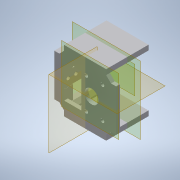
# Autodesk Inventor part: 30_Cube_Z_Focus_NEMA8_captive_base_v0
Saved by Autodesk Inventor 2022 (Build 260153000, 153)
## iProperties
Created: 2021-04-25
Part Number: 30_Cube_Z_Focus_NEMA8_captive_base_v0
Material: Generic
Document SubType Name: Modeling
Designer: diederichbenedict
Density: 1 g/cm^3
Appearance: Smooth - White
Author: diederichbenedict
Autodesk Inventor part; units mm, degrees
ref_plane "Work Plane1" through (0, 0, 13.5808) normal (0, 0, -1) x (-1, 0, 0)
sketch "Sketch1" plane through (0, 0, 13.5808) normal (0, 0, -1) x (-1, 0, 0)
  line L0 (24.85, 16.87) -> (16.87, 16.87)
  line L1 (16.87, -16.87) -> (24.85, -16.87)
  line L2 (24.85, -16.87) -> (24.85, 16.87)
  line L3 (-16.87, 24.85) -> (16.87, 24.85)
  line L4 (16.87, 24.85) -> (16.87, 13.87)
  line L5 (16.87, 13.87) -> (-16.87, 13.87)
  line L6 (-16.87, 13.87) -> (-16.87, 24.85)
  line L7 (-16.87, 16.87) -> (-24.85, 16.87)
  line L8 (-24.85, 16.87) -> (-24.85, -16.87)
  line L9 (-24.85, -16.87) -> (-16.87, -16.87)
  line L10 (-16.87, -24.85) -> (16.87, -24.85)
  line L11 (16.87, -24.85) -> (16.87, -13.87)
  line L12 (16.87, -13.87) -> (-16.87, -13.87)
  line L13 (-16.87, -13.87) -> (-16.87, -24.85)
  circle A0 centre (-22.53, 11.5) radius 1.025 construction
  circle A1 centre (-22.53, -11.5) radius 1.025 construction
  line L14 (-11.03, -14.1) -> (-11.03, -12.75) construction
  arc A2 (-11.03, 12.75) -> (-11.03, -12.75) centre (-11.03, 0) ccw construction
  line L15 (-11.03, 12.75) -> (-11.03, 14.1) construction
  line L16 (-11.03, 14.1) -> (-22.53, 14.1) construction
  arc A3 (-22.53, 14.1) -> (-25.13, 11.5) centre (-22.53, 11.5) ccw construction
  line L17 (-25.13, 11.5) -> (-25.13, -11.5) construction
  arc A4 (-25.13, -11.5) -> (-22.53, -14.1) centre (-22.53, -11.5) ccw construction
  line L18 (-22.53, -14.1) -> (-11.03, -14.1) construction
  circle A5 centre (-11.03, 0) radius 12.75 construction
  circle A6 centre (0.47, 11.5) radius 1.025 construction
  circle A7 centre (0.47, -11.5) radius 1.025 construction
  circle A8 centre (-22.53, -11.5) radius 1.025 construction
  circle A9 centre (-22.53, 11.5) radius 1.025 construction
  line L19 (-22.53, -14.1) -> (0.47, -14.1) construction
  arc A10 (-25.13, -11.5) -> (-22.53, -14.1) centre (-22.53, -11.5) ccw construction
  line L20 (-25.13, 11.5) -> (-25.13, -11.5) construction
  arc A11 (-22.53, 14.1) -> (-25.13, 11.5) centre (-22.53, 11.5) ccw construction
  line L21 (0.47, 14.1) -> (-22.53, 14.1) construction
  arc A12 (3.07, 11.5) -> (0.47, 14.1) centre (0.47, 11.5) ccw construction
  line L22 (3.07, -11.5) -> (3.07, 11.5) construction
  arc A13 (0.47, -14.1) -> (3.07, -11.5) centre (0.47, -11.5) ccw construction
  line L23 (-16.87, 13.87) -> (3.07, 13.87)
  line L24 (3.07, 13.87) -> (3.07, -13.87)
  line L25 (3.07, -13.87) -> (-16.87, -13.87)
  line L26 (16.87, 6.05) -> (16.8476, 6.05)
  line L27 (16.8476, 6.05) -> (16.8476, -6.05)
  line L28 (16.8476, -6.05) -> (16.87, -6.05)
  line L29 (16.87, -6.05) -> (16.87, -4.7)
  line L30 (16.87, 4.7) -> (16.87, 6.05)
  line L31 (16.87, 16.87) -> (16.87, 6.05)
  line L32 (16.87, -6.05) -> (16.87, -16.87)
  line L33 (5.6476, 13.2) -> (13.4476, 13.2) projected
  line L34 (13.4476, -13.2) -> (5.6476, -13.2) projected
  circle A14 centre (-4.7031, 0) radius 7 construction
  circle A15 centre (-4.7031, 0) radius 4 construction
  point P0 (0, 0)
  point P1 (16.87, 16.87)
  point P2 (3.07, 13.87)
  point P3 (3.07, 13.87)
  point P4 (-16.87, -16.87)
  dimension "d6" = 3
  dimension "d7" = 3
  dimension "d140" = 8
  constraints: 48 end point, 12 parallel, 7 perpendicular, 6 horizontal, 6 point on line, 2 centre point, 1 coincident, 2 other
  measures "d6" distance between parallel lines of L7 L5
  measures "d7" distance between parallel lines of L9 L12
  measures "d140" diameter of A15
extrude "Extrusion1" add sketch "Sketch1" along normal blind 3 contours L2 L1 L11 L32 L28 L27 L26 L31 L4 L0 | L4 L5 L6 L3 | L11 L10 L13 L12 | L24 L12 L13 L9 L8 L7 L6 L5
chamfer "Chamfer1" distance 3.9 angle 45 4 edges at (-16.87, -16.87, 12.0808) (16.87, -16.87, 12.0808) (16.87, 16.87, 12.0808) (-16.87, 16.87, 12.0808)
sketch "Sketch2" plane through (0, 0, 10.5808) normal (0, 0, -1) x (-1, 0, 0)
  line L0 (3.07, 13.87) -> (16.87, 13.87) projected
  line L1 (16.87, -13.87) -> (3.07, -13.87) projected
  line L2 (-16.87, -20.77) -> (-16.87, -24.85) construction
  line L3 (-16.87, -24.85) -> (16.87, -24.85) construction
  line L4 (16.87, -6.05) -> (16.87, -13.87) projected
  line L5 (16.87, 20.77) -> (16.87, 24.85) construction
  line L6 (16.87, 24.85) -> (-16.87, 24.85) construction
  line L7 (-16.87, 24.85) -> (-16.87, 20.77) construction
  line L8 (-13.8689, -21.8489) -> (-13.8689, -19.5269)
  line L9 (-13.8689, -19.5269) -> (-19.5269, -13.8689)
  line L10 (-19.5269, -13.8689) -> (-21.8489, -13.8689)
  line L11 (-21.8489, 13.8689) -> (-19.5269, 13.8689)
  line L12 (-19.5269, 13.8689) -> (-13.8689, 19.5269)
  line L13 (-13.8689, 19.5269) -> (-13.8689, 21.8489)
  line L14 (-13.8689, 21.8489) -> (-13.8689, 24.85)
  line L15 (-21.8489, 13.8689) -> (-24.85, 13.8689)
  line L16 (-21.8489, -13.8689) -> (-24.85, -13.8689)
  line L17 (-13.8689, -21.8489) -> (-13.8689, -24.85)
  line L18 (-11.5469, -21.8489) -> (-13.8689, -21.8489)
  line L19 (-21.8489, -13.8689) -> (-21.8489, -11.5469)
  line L20 (-21.8489, 11.5469) -> (-21.8489, 13.8689)
  line L21 (-13.8689, 21.8489) -> (-11.5469, 21.8489)
  line L22 (16.87, 13.87) -> (16.87, 6.05) projected
  line L23 (16.87, 6.05) -> (16.8476, 6.05) projected
  line L24 (16.8476, 6.05) -> (16.8476, -6.05) projected
  line L25 (16.8476, -6.05) -> (16.87, -6.05) projected
  line L26 (20.77, -16.87) -> (24.85, -16.87) construction
  line L27 (24.85, -16.87) -> (24.85, 16.87) construction
  line L28 (24.85, 16.87) -> (20.77, 16.87) construction
  line L29 (16.87, 20.77) -> (20.77, 16.87) construction
  line L30 (16.87, -24.85) -> (16.87, -20.77) construction
  line L31 (20.77, -16.87) -> (16.87, -20.77) construction
  line L32 (-13.87, 21.85) -> (13.87, 21.85) construction
  line L33 (13.87, 21.85) -> (13.87, 19.5274) construction
  line L34 (13.87, 19.5274) -> (19.5274, 13.87) construction
  line L35 (19.5274, 13.87) -> (21.85, 13.87) construction
  line L36 (21.85, 13.87) -> (21.85, -13.87) construction
  line L37 (21.85, -13.87) -> (19.5274, -13.87) construction
  line L38 (19.5274, -13.87) -> (13.87, -19.5274) construction
  line L39 (13.87, -19.5274) -> (13.87, -21.85) construction
  line L40 (13.87, -21.85) -> (-13.87, -21.85) construction
  line L41 (-13.87, -21.85) -> (-13.87, -19.5274) construction
  line L42 (-13.87, -19.5274) -> (-19.5274, -13.87) construction
  line L43 (-19.5274, -13.87) -> (-21.85, -13.87) construction
  line L44 (-21.85, -13.87) -> (-21.85, 13.87) construction
  line L45 (-21.85, 13.87) -> (-19.5274, 13.87) construction
  line L46 (-19.5274, 13.87) -> (-13.87, 19.5274) construction
  line L47 (-13.87, 19.5274) -> (-13.87, 21.85) construction
  line L48 (16.87, 24.85) -> (-16.87, 24.85) projected
  line L49 (13.87, 24.85) -> (13.87, 19.5274)
  line L50 (13.87, 19.5274) -> (19.5274, 13.87)
  line L51 (19.5274, 13.87) -> (24.85, 13.87)
  line L52 (24.85, -16.87) -> (24.85, 16.87) projected
  line L53 (24.85, -13.87) -> (19.5274, -13.87)
  line L54 (19.5274, -13.87) -> (13.87, -19.5274)
  line L55 (-16.87, -24.85) -> (16.87, -24.85) projected
  line L56 (13.87, -24.85) -> (13.87, -19.5274)
  line L57 (16.87, 24.85) -> (-16.87, 24.85) projected
  line L58 (13.87, 24.85) -> (16.87, 24.85)
  line L59 (16.87, 24.85) -> (16.87, 20.77)
  line L60 (16.87, 20.77) -> (20.77, 16.87)
  line L61 (24.85, 16.87) -> (20.77, 16.87) projected
  line L62 (24.85, 16.87) -> (20.77, 16.87)
  line L63 (24.85, -16.87) -> (24.85, 16.87) projected
  line L64 (24.85, 16.87) -> (24.85, 13.87)
  line L65 (24.85, -13.87) -> (24.85, -16.87)
  line L66 (24.85, -16.87) -> (20.77, -16.87)
  line L67 (20.77, -16.87) -> (16.87, -20.77)
  line L68 (16.87, -24.85) -> (16.87, -20.77) projected
  line L69 (16.87, -24.85) -> (16.87, -20.77)
  line L70 (16.87, -20.77) -> (16.87, -24.85)
  line L71 (16.87, -24.85) -> (-16.87, -24.85) projected
  line L72 (13.87, -24.85) -> (16.87, -24.85)
  line L73 (3.07, -13.87) -> (3.07, 13.87) projected
  line L74 (-20.77, 16.87) -> (-24.85, 16.87) projected
  line L75 (-24.85, 16.87) -> (-24.85, -16.87) projected
  line L76 (-24.85, -16.87) -> (-20.77, -16.87) projected
  line L77 (-16.87, -20.77) -> (-20.77, -16.87) projected
  line L78 (-20.77, 16.87) -> (-16.87, 20.77) projected
  point P0 (0, 0)
  dimension "d115" = 3
  constraints: 94 end point, 14 point on line, 6 collinear, 5 perpendicular, 1 horizontal, 1 vertical, 9 other
  measures "d115" distance between parallel lines of L6 L32
ref_plane "Work Plane2" through (-16.97, -24.85, 34.1) normal (0, 0, -1) x (0, 1, 0)
extrude "Extrusion2" add sketch "Sketch2" along normal blind 31.5 contours L56 L54 L53 L52 L66 L67 L68 L55 | L51 L50 L49 L48 L59 L60 L61 L52
sketch "Sketch4" plane through (-24.85, -16.87, 13.5808) normal (-1, 0, 0) x (0, 0, 1)
  line L0 (37.9, 11.3739) -> (37.9, 18.453) construction
  line L1 (23.6194, 18.453) -> (37.9, 18.453) construction
  arc A0 (22.1806, 18.453) -> (23.6194, 18.453) centre (22.9, 16.8577) ccw construction
  line L2 (-1.3806, 18.453) -> (22.1806, 18.453) construction
  arc A1 (-2.8194, 18.453) -> (-1.3806, 18.453) centre (-2.1, 16.8577) ccw construction
  line L3 (-31.3806, 18.453) -> (-2.8194, 18.453) construction
  arc A2 (-32.8194, 18.453) -> (-31.3806, 18.453) centre (-32.1, 16.8577) ccw construction
  line L4 (-42.1, 18.453) -> (-32.8194, 18.453) construction
  line L5 (-42.1, 11.3739) -> (-42.1, 18.453) construction
  line L6 (-42.1, 11.3739) -> (37.9, 11.3739) construction
  line L7 (37.9, 19.2506) -> (37.9, 22.3415) construction
  line L8 (-42.1, 22.3415) -> (37.9, 22.3415) construction
  line L9 (-42.1, 19.2506) -> (-42.1, 22.3415) construction
  line L10 (-42.1, 19.2506) -> (37.9, 19.2506) construction
  line L11 (-3, 3) -> (-3, 30.74) construction
  line L12 (-34.1, 33.84) -> (-34.1, -5.98) construction
  line L13 (-3, 11.3739) -> (-34.1, 11.3739)
  line L14 (-34.1, 11.3739) -> (-34.1, 22.3415)
  line L15 (-34.1, 22.3415) -> (-3, 22.3415)
  line L16 (-3, 22.3415) -> (-3, 11.3739)
  line L17 (-34.1, 11.3739) -> (-32.1, 11.3739)
  line L18 (-32.1, 11.3739) -> (-32.1, 3.0011)
  line L19 (-32.1, 3.0011) -> (-34.1, 3.0011)
  line L20 (-34.1, 3.0011) -> (-34.1, 11.3739)
  line L21 (-34.1, 22.3415) -> (-32.1, 22.3415)
  line L22 (-32.1, 22.3415) -> (-32.1, 30.7389)
  line L23 (-32.1, 30.7389) -> (-34.1, 30.7389)
  line L24 (-34.1, 30.7389) -> (-34.1, 22.3415)
  point P0 (-13.5808, 16.87)
  point P1 (-3, 3.0011)
  point P2 (-3, 30.7389)
  point P3 (-3, 33.74)
  point P4 (-3, 31.418)
  point P5 (-3, 0)
  dimension "d24" = 2
  constraints: 24 end point, 6 parallel, 5 point on line, 3 horizontal, 3 perpendicular
  measures "d24" distance of L18.end L19.end
ref_plane "Work Plane3" through (16.97, -5.4961, -37.9) normal (1, 0, 0) x (0, 1, 0)
extrude "Extrusion4" add sketch "Sketch4" against normal blind 7.88 contours L13 L14 L15 L16
sketch "Sketch5" plane through (-24.85, -16.87, 13.5808) normal (-1, 0, 0) x (0, 0, 1)
  circle A0 centre (-32.1, 16.87) radius 1.4
  circle A1 centre (-3.4423, 16.87) radius 1.4
  line L0 (0, -7.98) -> (-34.5, -7.98) projected
  line L1 (0, 41.72) -> (-34.5, 41.72) projected
  line L2 (0, -7.98) -> (-34.5, -7.98) projected
  point P0 (-13.5808, 16.87)
  dimension "d25" = 2.8
  dimension "d26" = 2.8
  dimension "d86" = 49.7
  dimension "d87" = 24.85
  dimension "d88" = 0
  constraints: 2 centre point
  measures "d25" diameter of A0
  measures "d26" diameter of A1
  measures "d86" distance between parallel lines of L1 L2
  measures "d87" distance from line of A0.centre L1
  measures "d88" vertical distance of A1.centre A0.centre
extrude "Extrusion5" cut sketch "Sketch5" against normal blind 10
pattern_linear "Rectangular Pattern1" count 5 spacing 6.25 along (0, 0, -1) of "Extrusion5"
ref_plane "Work Plane4" through (-25.03, -12.97, -12) normal (0, 0, 1) x (1, 0, 0)
sketch "Sketch12" plane through (-24.85, -16.87, 13.5808) normal (-1, 0, 0) x (0, 0, 1)
  ellipse E0 centre (-17.053, 16.87) end of major axis (-32.053, 16.87) minor radius 10.6066 projected
  circle A0 centre (-32.1, 16.87) radius 1.4 projected
  circle A1 centre (-22.1923, 16.87) radius 1.4 projected
  circle A2 centre (-15.9423, 16.87) radius 1.4 projected
  circle A3 centre (-9.6923, 16.87) radius 1.4 projected
  circle A4 centre (-3.4423, 16.87) radius 1.4 projected
  circle A5 centre (-28.4423, 16.87) radius 1.4 projected
  point P0 (-13.5808, 16.87)
  constraints: 1 other
hole "Hole2" at (-24.85, 0, -8.6115) at (-24.85, 0, 3.8885) at (-24.85, 0, 10.1385) at (-24.85, 0, -2.3615) at (-24.85, 0, -14.8615) direction (1, 0, 0) diameter 2.8 depth 8 tip angle 118 counterbore diameter 6 counterbore depth 3
ref_plane "Work Plane6" through (0, 0, -22) normal (0, 0, -1) x (-1, 0, 0)
ref_plane "Work Plane5" through (-16.97, -16.97, 0) normal (0, 0, 1) x (1, 0, 0)
ref_plane "Work Plane7" through (0, -16.87, 13.5808) normal (1, 0, 0) x (0, 0, -1)
ref_plane "Work Plane8" through (16.87, 0, 13.5808) normal (0, 1, 0) x (-1, 0, 0)
sketch "Skizze18" plane through (-24.85, -16.87, 13.5808) normal (-1, 0, 0) x (0, 0, 1)
  line L0 (0, 0) -> (-34.5, 0) projected
  line L1 (0, 0) -> (0, 33.74) projected
  line L2 (0, 33.74) -> (-34.5, 33.74) projected
  arc A0 (-31.2335, 15.7704) -> (-31.2335, 17.9696) centre (-28.4423, 16.87) ccw projected
  arc A1 (-31.2335, 17.9696) -> (-31.2335, 15.7704) centre (-32.1, 16.87) ccw projected
  circle A2 centre (-3.4423, 16.87) radius 3 projected
  circle A3 centre (-22.1923, 16.87) radius 3 projected
  circle A4 centre (-9.6923, 16.87) radius 3 projected
  circle A5 centre (-15.9423, 16.87) radius 3 projected
  line L3 (-3, 30.7389) -> (-34.5, 30.7389) projected
  line L4 (-34.1, 30.7389) -> (-3, 30.7389)
  line L5 (-3, 30.7389) -> (-3, 33.74)
  line L6 (-3, 33.74) -> (-34.1, 33.74)
  line L7 (-34.1, 33.74) -> (-34.1, 30.7389)
  line L8 (-3, 3.0011) -> (-34.5, 3.0011) projected
  line L9 (0, 0) -> (-34.5, 0) projected
  line L10 (-3, 3.0011) -> (-34.1, 3.0011)
  line L11 (-34.1, 3.0011) -> (-34.1, 0)
  line L12 (-34.1, 0) -> (-3, 0)
  line L13 (-3, 0) -> (-3, 3.0011)
  line L14 (-3, 3) -> (-3, 11.3739) projected
  line L15 (-34.1, 22.3415) -> (-3, 22.3415) projected
  line L16 (-34.1, 11.3739) -> (-34.1, 22.3415) projected
  line L17 (-3, 11.3739) -> (-34.1, 11.3739) projected
  line L18 (-3, 22.3415) -> (-3, 30.74) projected
  line L19 (-34.5, 30.74) -> (-34.5, 33.74) projected
  line L20 (-3, 30.74) -> (-34.5, 30.74) projected
  line L21 (-3, 3) -> (-34.5, 3) projected
  line L22 (-34.5, 0) -> (-34.5, 3) projected
  point P0 (-13.5808, 16.87)
  point P1 (-35.1, 0)
  point P2 (-34.1, 3.0011)
  point P3 (-3, 0)
  point P4 (-34.1, 0)
  constraints: 16 end point, 4 parallel, 3 point on line, 2 horizontal, 2 perpendicular
extrude "Extrusion14" cut sketch "Skizze18" against normal blind 10 contours L0 L11 L8 L13 | L5 L3 L7 L2
sketch "Skizze19" plane through (0, 0, 13.5808) normal (0, 0, 1) x (1, 0, 0)
  line L0 (-34.5437, 37.7032) -> (40.2308, 37.7032)
  line L1 (40.2308, 37.7032) -> (40.2308, -45.0753)
  line L2 (40.2308, -45.0753) -> (-34.5437, -45.0753)
  line L3 (-34.5437, -45.0753) -> (-34.5437, 37.7032)
  point P0 (0, 0)
  constraints: 8 end point, 2 parallel, 1 horizontal, 1 perpendicular
extrude "Extrusion15" cut sketch "Skizze19" against normal blind 34 keep common part
sketch "Skizze20" plane through (0, 0, 13.5808) normal (0, 0, 1) x (1, 0, 0)
  line L0 (-16.87, 24.85) -> (16.87, 24.85) projected
  line L1 (-16.87, -24.85) -> (16.87, -24.85) projected
  line L2 (16.87, 24.85) -> (16.87, 20.77) projected
  line L3 (-16.87, 24.85) -> (16.87, 24.85)
  line L4 (16.87, 24.85) -> (16.87, 20.85)
  line L5 (16.87, 20.85) -> (-16.87, 20.85)
  line L6 (-16.87, 20.85) -> (-16.87, 24.85)
  line L7 (-16.87, -13.87) -> (-16.87, -13.87) projected
  line L8 (-16.87, -24.85) -> (16.87, -24.85)
  line L9 (16.87, -24.85) -> (16.87, -20.85)
  line L10 (16.87, -20.85) -> (-16.87, -20.85)
  line L11 (-16.87, -20.85) -> (-16.87, -24.85)
  point P0 (0, 0)
  point P1 (-16.87, -20.77)
  point P2 (16.87, -24.85)
  point P3 (-16.87, -20.85)
  point P4 (16.87, 13.87)
  dimension "d104" = 4
  dimension "d105" = 4
  constraints: 16 end point, 4 parallel, 2 horizontal, 2 perpendicular, 2 point on line, 1 other
  measures "d104" distance of L3.end L4.end
  measures "d105" distance of L9.end L8.end
extrude "Extrusion16" add sketch "Skizze20" against normal blind 34
sketch "Skizze25" plane through (0, 0, 10.5808) normal (0, 0, -1) x (-1, 0, 0)
  line L0 (13.87, 20.85) -> (-16.87, 20.85) projected
  line L1 (-16.87, 20.85) -> (-16.87, 20.77) projected
  line L2 (-20.77, 16.87) -> (-16.87, 20.77) projected
  line L3 (-20.77, 16.87) -> (-24.85, 16.87) projected
  line L4 (-24.85, 16.87) -> (-24.85, -16.87) projected
  line L5 (-24.85, -16.87) -> (-20.77, -16.87) projected
  line L6 (-16.87, -20.77) -> (-20.77, -16.87) projected
  line L7 (-16.87, -20.77) -> (-16.87, -20.85) projected
  line L8 (-16.87, -20.85) -> (13.87, -20.85) projected
  line L9 (13.87, -20.85) -> (13.87, -19.5274) projected
  line L10 (13.87, -19.5274) -> (16.5274, -16.87) projected
  line L11 (20.77, -16.87) -> (16.5274, -16.87) projected
  line L12 (24.85, -16.87) -> (20.77, -16.87) projected
  line L13 (24.85, -16.87) -> (24.85, -5.4961) projected
  line L14 (24.85, -5.4961) -> (16.97, -5.4961) projected
  line L15 (16.8476, 6.05) -> (16.8476, 1.3283) projected
  line L16 (16.8476, -6.05) -> (16.87, -6.05) projected
  line L17 (16.87, -6.05) -> (16.87, -13.87) projected
  line L18 (16.87, -13.87) -> (3.07, -13.87) projected
  line L19 (3.07, -13.87) -> (3.07, 13.87) projected
  line L20 (3.07, 13.87) -> (16.87, 13.87) projected
  line L21 (16.87, 13.87) -> (16.87, 6.05) projected
  line L22 (16.87, 6.05) -> (16.8476, 6.05) projected
  line L23 (16.8476, -1.3283) -> (16.8476, -6.05) projected
  line L24 (16.97, 5.4715) -> (24.85, 5.4715) projected
  line L25 (24.85, 5.4715) -> (24.85, 16.87) projected
  line L26 (20.77, 16.87) -> (24.85, 16.87) projected
  line L27 (20.77, 16.87) -> (16.5274, 16.87) projected
  line L28 (16.5274, 16.87) -> (13.87, 19.5274) projected
  line L29 (13.87, 19.5274) -> (13.87, 20.85) projected
  line L30 (16.87, 13.87) -> (16.87, 16.87)
  line L31 (16.87, -6.05) -> (16.87, -13.87) projected
  line L32 (16.87, -13.87) -> (16.87, -16.87)
  line L33 (20.77, -16.87) -> (16.5274, -16.87) projected
  line L34 (16.97, -5.4961) -> (16.97, -1.3283) projected
  line L35 (16.97, -1.3283) -> (16.8476, -1.3283) projected
  line L36 (16.8476, 1.3283) -> (16.97, 1.3283) projected
  line L37 (16.97, 1.3283) -> (16.97, 5.4715) projected
  point P0 (0, 0)
  constraints: 4 end point, 3 point on line, 1 vertical
extrude "Extrusion21" add sketch "Skizze25" along normal blind 4 contours L27 L26 L25 L24 L37 L36 L15 L22 L21 L30 | L17 L16 L23 L35 L34 L14 L13 L12 L11 L32
ref_plane "Arbeitsebene9" through (0, 0, -3.4192) normal (0, 0, -1) x (-1, 0, 0)
sketch "Skizze29" plane through (0, 0, 13.5808) normal (0, 0, 1) x (1, 0, 0)
  circle A0 centre (5.0933, 0) radius 5.5
  circle A1 centre (5.2366, 0) radius 2.75 projected
  circle A2 centre (5.2366, 0) radius 8 projected
  point P0 (0, 0)
  dimension "d152" = 11
  constraints: 1 centre point
  measures "d152" diameter of A0
extrude "Extrusion25" cut sketch "Skizze29" against normal blind 10 contours A0 | A1
sketch "Skizze31" plane through (0, 0, 10.5808) normal (0, 0, -1) x (-1, 0, 0)
  circle A0 centre (-5.0933, 0) radius 5.5 projected
  line L0 (16.87, -16.87) -> (16.87, -13.87) projected
  line L1 (16.87, -13.87) -> (3.07, -13.87) projected
  line L2 (3.07, -13.87) -> (3.07, 13.87) projected
  line L3 (3.07, 13.87) -> (16.87, 13.87) projected
  line L4 (16.87, 13.87) -> (16.87, 16.87) projected
  line L5 (16.87, 16.87) -> (16.5274, 16.87) projected
  line L6 (16.5274, 16.87) -> (13.87, 19.5274) projected
  line L7 (13.87, 19.5274) -> (13.87, 20.85) projected
  line L8 (13.87, 20.85) -> (-16.87, 20.85) projected
  line L9 (-16.87, 20.85) -> (-16.87, 20.77) projected
  line L10 (-20.77, 16.87) -> (-16.87, 20.77) projected
  line L11 (-20.77, 16.87) -> (-24.85, 16.87) projected
  line L12 (-24.85, 16.87) -> (-24.85, -16.87) projected
  line L13 (-24.85, -16.87) -> (-20.77, -16.87) projected
  line L14 (-16.87, -20.77) -> (-20.77, -16.87) projected
  line L15 (-16.87, -20.77) -> (-16.87, -20.85) projected
  line L16 (-16.87, -20.85) -> (13.87, -20.85) projected
  line L17 (13.87, -20.85) -> (13.87, -19.5274) projected
  line L18 (13.87, -19.5274) -> (16.5274, -16.87) projected
  line L19 (16.87, -16.87) -> (16.5274, -16.87) projected
  line L20 (-13.85, -12.5) -> (-0.85, -12.5)
  line L21 (-0.85, -12.5) -> (-0.85, 12.5)
  line L22 (-0.85, 12.5) -> (-13.85, 12.5)
  line L23 (-13.85, 12.5) -> (-13.85, -12.5)
  line L24 (-13.85, -12.5) -> (-0.85, 12.5) construction
  line L25 (-0.85, -12.5) -> (-13.85, 12.5) construction
  point P0 (0, 0)
  point P1 (-7.35, 0)
  dimension "d153" = 13
  dimension "d154" = 25
  dimension "d155" = 11
  constraints: 12 end point, 2 midpoint, 2 parallel, 1 horizontal, 1 perpendicular
  measures "d153" distance of L22.end L21.end
  measures "d154" distance of L21.end L20.end
  measures "d155" distance between parallel lines of L23 L12
hole "Bohrung4" at (0.85, 12.5, 10.5808) at (13.85, 12.5, 10.5808) at (13.85, -12.5, 10.5808) at (0.85, -12.5, 10.5808) direction (0, 0, 1) diameter 3 end through all
body "Solid1"
